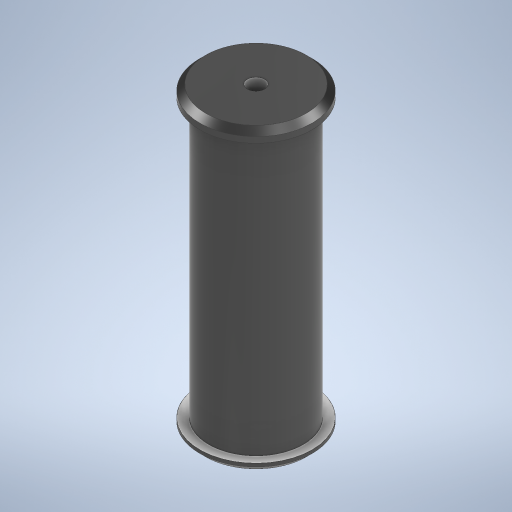
# Autodesk Inventor part: roda
Saved by Autodesk Inventor 2023 (Build 270158000, 158)
## iProperties
Created: 2023-08-08
Part Number: roda
Material: Genérico
Document SubType Name: Modeling
Designer: azeve
Density: 1 g/cm^3
Appearance: Padrão
Author: azeve
Autodesk Inventor part; units mm, degrees
ref_plane "YZ Plane" through (0, 0, 0) normal (1, 0, 0) x (0, 1, 0)
ref_plane "XZ Plane" through (0, 0, 0) normal (0, 1, 0) x (-1, 0, 0)
ref_plane "XY Plane" through (0, 0, 0) normal (0, 0, 1) x (1, 0, 0)
sketch "Esboço1" plane through (0, 0, 0) normal (0, 0, 1) x (1, 0, 0)
  line L0 (0, 0) -> (0, 57)
  line L1 (8.2179, 1.5639) -> (9.7832, 1.5639)
  line L2 (9.7832, 1.5639) -> (9.7832, 0)
  line L3 (7.3887, 0.7346) -> (7.3887, 39.3227)
  line L4 (7.3887, 0.7346) -> (7.3887, 0)
  line L5 (7.3887, 0) -> (9.7832, 0)
  line L6 (9.7832, 0) -> (7.3887, 0)
  line L7 (0.8292, 0) -> (0, 0)
  line L8 (0, 42.2247) -> (0, 57)
  line L9 (0, 42.2247) -> (0, 39.7247)
  line L10 (0, 55.3122) -> (0, 52.8122)
  line L11 (8.2179, 49.9102) -> (8.2179, 1.5639)
  line L12 (0, 42.2247) -> (0, 39.3227)
  line L13 (0, 39.3227) -> (7.3887, 39.3227)
  line L14 (0, 52.8122) -> (0, 49.9102)
  line L15 (8.2179, 49.9102) -> (9.7832, 49.9102)
  line L16 (9.7832, 49.9102) -> (9.7832, 51.9102)
  line L17 (9.7832, 51.9102) -> (0, 51.9102)
  constraints: 36 end point, 7 point on line, 5 perpendicular, 3 vertical, 2 horizontal
revolve "Revolução1" add sketch "Esboço1" angle 360 about axis through (0, 0, 0) along (0, 1, 0)
chamfer "Chanfro2" distance 1 angle 45 1 edges at (-9.7832, 0, 0)
chamfer "Chanfro4" distance 1 angle 45 1 edges at (-9.7832, 51.9102, 0)
sketch "Esboço4" plane through (0, 51.9102, 0) normal (0, 1, 0) x (1, 0, 0)
  circle A0 centre (0, 0) radius 8.7832 projected
  constraints: 1 coincident
hole "Furo2" at (0, 51.9102, 0) direction (0, -1, 0) diameter 3 depth 19.499 tip angle 118
